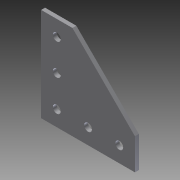
# Autodesk Inventor part: common angle bracket
Saved by Autodesk Inventor 2011 SP1 (Build 150282100, 282)
## iProperties
Created: 2012-01-20
Part Number: common angle bracket
Document SubType Name: Modeling
Designer: Christopher
Density: 1 g/cm^3
Author: Christopher
Autodesk Inventor part; units mm, degrees
ref_plane "YZ Plane" through (0, 0, 0) normal (1, 0, 0) x (0, 1, 0)
ref_plane "XZ Plane" through (0, 0, 0) normal (0, 1, 0) x (-1, 0, 0)
ref_plane "XY Plane" through (0, 0, 0) normal (0, 0, 1) x (1, 0, 0)
sketch "Sketch1" plane through (0, 0, 0) normal (0, 0, 1) x (1, 0, 0)
  line L0 (0, 0) -> (0, 76.2)
  line L1 (0, 76.2) -> (25.4, 76.2)
  line L2 (25.4, 76.2) -> (76.2, 25.4)
  line L3 (76.2, 25.4) -> (76.2, 0)
  line L4 (76.2, 0) -> (0, 0)
  point P0 (12.7, 63.5)
  point P1 (12.7, 38.1)
  point P2 (12.7, 12.7)
  point P3 (38.1, 12.7)
  point P4 (63.5, 12.7)
  dimension "d0" = 76.2
  dimension "d1" = 76.2
  dimension "d2" = 25.4
  dimension "d3" = 25.4
  dimension "d4" = 12.7
  dimension "d5" = 12.7
  dimension "d6" = 25.4
  dimension "d7" = 25.4
  dimension "d8" = 25.4
  dimension "d9" = 25.4
  constraints: 10 end point, 2 horizontal alignment, 2 parallel, 2 vertical alignment, 1 perpendicular, 1 vertical
  measures "d0" distance of L3.end L0.start
  measures "d1" distance of L0.start L0.end
  measures "d2" distance of L0.end L1.end
  measures "d3" distance of L2.end L3.end
  measures "d4" distance from line of L4 point (63.5, 12.7)
  measures "d5" distance from line of L0 point (12.7, 63.5)
  measures "d6" distance of point (12.7, 12.7) point (38.1, 12.7)
  measures "d7" distance of point (63.5, 12.7) point (38.1, 12.7)
  measures "d8" distance of point (12.7, 12.7) point (12.7, 38.1)
  measures "d9" distance of point (12.7, 63.5) point (12.7, 38.1)
extrude "Extrusion1" add sketch "Sketch1" against normal blind 3.175
hole "Hole1" at (12.7, 63.5, 0) at (12.7, 38.1, 0) at (12.7, 12.7, 0) at (38.1, 12.7, 0) at (63.5, 12.7, 0) direction (0, 0, -1) diameter 6.35 depth 25.4 tip angle 118
body "Solid1"
